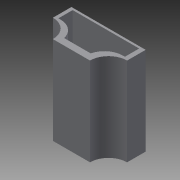
# Autodesk Inventor part: USB-slot
Saved by Autodesk Inventor 2015 (Build 190159000, 159)
## iProperties
Created: 2015-09-08
Part Number: USB-slot
Material: Generic
Document SubType Name: Modeling
Designer: david
Density: 1 g/cm^3
Appearance: Default
Author: david
Autodesk Inventor part; units mm, degrees
ref_plane "YZ Plane" through (0, 0, 0) normal (1, 0, 0) x (0, 1, 0)
ref_plane "XZ Plane" through (0, 0, 0) normal (0, 1, 0) x (-1, 0, 0)
ref_plane "XY Plane" through (0, 0, 0) normal (0, 0, 1) x (1, 0, 0)
sketch "Sketch1" plane through (0, 0, 0) normal (0, 1, 0) x (-1, 0, 0)
  line L0 (-4, 4.75) -> (4, 4.75)
  line L1 (4, 4.75) -> (4, -4.75)
  line L2 (4, -4.75) -> (-4, -4.75)
  line L3 (-4, -4.75) -> (-4, 4.75)
  line L4 (-4, 4.75) -> (4, -4.75) construction
  line L5 (4, 4.75) -> (-4, -4.75) construction
  point P0 (0, 0)
  dimension "d0" = 8
  dimension "d1" = 9.5
  constraints: 12 end point, 2 midpoint, 2 parallel, 1 horizontal, 1 perpendicular
  measures "d0" distance of L1.end L2.end
  measures "d1" distance of L0.end L1.end
extrude "Extrusion1" add sketch "Sketch1" along normal blind 4
sketch "Sketch2" plane through (-4, 0, 4.75) normal (0, 0, 1) x (1, 0, 0)
  circle A0 centre (0, 0) radius 2
  circle A1 centre (8, 0) radius 2
  point P0 (4, 0)
  dimension "d4" = 4
  dimension "d5" = 4
  constraints: 2 centre point
  measures "d4" diameter of A0
  measures "d5" diameter of A1
extrude "Extrusion2" cut sketch "Sketch2" against normal blind 10
sketch "Sketch3" plane through (-4, 4, 4.75) normal (0, 0, 1) x (1, 0, 0)
  line L0 (0.3545, -0.2253) -> (7.5248, -0.2253)
  line L1 (7.5248, -0.2253) -> (7.5248, -1.7593)
  line L2 (7.5248, -1.7593) -> (0.3545, -1.7593)
  line L3 (0.3545, -1.7593) -> (0.3545, -0.2253)
  line L4 (2.5091, -3.2933) -> (5.3703, -3.2933)
  line L5 (5.3703, -3.2933) -> (5.3703, -0.2253)
  line L6 (5.3703, -0.2253) -> (2.5091, -0.2253)
  line L7 (2.5091, -0.2253) -> (2.5091, -3.2933)
  line L8 (2.5091, -3.2933) -> (5.3703, -0.2253) construction
  line L9 (5.3703, -3.2933) -> (2.5091, -0.2253) construction
  point P0 (4, -4)
  point P1 (3.9397, -1.7593)
  constraints: 20 end point, 4 parallel, 3 midpoint, 2 horizontal, 2 perpendicular, 1 point on line
extrude "Extrusion3" cut sketch "Sketch3" against normal blind 8
fillet "Fillet1" radius 2 2 edges at (-1.4909, 2.2407, 0.75) (1.3703, 2.2407, 0.75)
body "Solid1"
